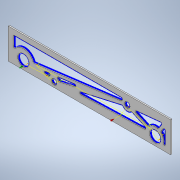
# Autodesk Inventor part: Right right side
Saved by Autodesk Inventor 2021 (Build 250183000, 183)
## iProperties
Created: 2020-09-20
Part Number: Right right side
Material: Generic
Document SubType Name: Modeling
Designer: deli
Density: 1 g/cm^3
Appearance: Default
Author: deli
Autodesk Inventor part; units mm, degrees
ref_plane "YZ Plane" through (0, 0, 0) normal (1, 0, 0) x (0, 1, 0)
ref_plane "XZ Plane" through (0, 0, 0) normal (0, 1, 0) x (-1, 0, 0)
ref_plane "XY Plane" through (0, 0, 0) normal (0, 0, 1) x (1, 0, 0)
sketch "Sketch1" plane through (0, 0, 0) normal (0, 0, 1) x (1, 0, 0)
  line L0 (125.1151, 28.732) -> (166.2826, 33.9736)
  arc A0 (167.3819, 27.7268) -> (166.2826, 33.9736) centre (166.6836, 30.824) ccw
  line L1 (167.3819, 27.7268) -> (129.3518, 19.1523)
  arc A1 (126.0625, 20.4145) -> (129.3518, 19.1523) centre (128.6535, 22.2495) ccw
  arc A2 (126.0625, 20.4145) -> (123.528, 23.1069) centre (115.1699, 12.7) ccw
  arc A3 (125.1151, 28.732) -> (123.528, 23.1069) centre (125.5161, 25.5824) ccw
  line L2 (321.3346, 53.089) -> (381.486, 59.0906)
  arc A4 (384.529, 54.3066) -> (381.486, 59.0906) centre (381.8012, 55.9313) ccw
  line L3 (384.529, 54.3066) -> (377.4306, 42.3884)
  arc A5 (373.8567, 40.9528) -> (377.4306, 42.3884) centre (374.7028, 44.013) ccw
  arc A6 (373.8567, 40.9528) -> (352.4725, 34.4311) centre (368.3, 20.8534) ccw
  arc A7 (348.7058, 33.6279) -> (352.4725, 34.4311) centre (350.0627, 36.4983) ccw
  line L4 (348.7058, 33.6279) -> (320.2929, 47.0593)
  arc A8 (321.3346, 53.089) -> (320.2929, 47.0593) centre (321.6498, 49.9297) ccw
  arc A9 (388.6543, 16.3183) -> (390.525, 12.7) centre (391.7533, 15.6278) ccw
  arc A10 (388.6543, 16.3183) -> (383.3263, 35.3128) centre (368.3, 20.8534) ccw
  arc A11 (382.8862, 39.139) -> (383.3263, 35.3128) centre (385.6141, 37.5143) ccw
  line L5 (382.8862, 39.139) -> (387.7972, 47.3844)
  arc A12 (393.7, 45.7598) -> (387.7972, 47.3844) centre (390.525, 45.7598) ccw
  line L6 (393.7, 45.7598) -> (393.7, 15.875)
  arc A13 (390.525, 12.7) -> (393.7, 15.875) centre (390.525, 15.875) ccw
  line L7 (12.7, 38.8139) -> (12.7, 60.325)
  arc A14 (15.875, 63.5) -> (12.7, 60.325) centre (15.875, 60.325) ccw
  line L8 (15.875, 63.5) -> (282.9805, 63.5)
  arc A15 (285.9117, 59.1048) -> (282.9805, 63.5) centre (282.9805, 60.325) ccw
  arc A16 (285.9117, 59.1048) -> (285.3624, 57.5073) centre (298.2343, 53.975) ccw
  arc A17 (282.7016, 55.1979) -> (285.3624, 57.5073) centre (282.3006, 58.3475) ccw
  line L9 (282.7016, 55.1979) -> (65.3364, 27.5219)
  arc A18 (61.9536, 29.5806) -> (65.3364, 27.5219) centre (64.9353, 30.6715) ccw
  arc A19 (61.9536, 29.5806) -> (18.3444, 36.8183) centre (38.1, 20.8534) ccw
  arc A20 (12.7, 38.8139) -> (18.3444, 36.8183) centre (15.875, 38.8139) ccw
  arc A21 (341.9094, 23.18) -> (343.1641, 29.2238) centre (341.8072, 26.3534) ccw
  line L10 (341.9094, 23.18) -> (181.8296, 18.0238)
  arc A22 (181.0291, 24.2944) -> (181.8296, 18.0238) centre (181.7274, 21.1971) ccw
  line L11 (181.0291, 24.2944) -> (284.0524, 47.5227)
  arc A23 (287.3417, 46.2605) -> (284.0524, 47.5227) centre (284.7507, 44.4255) ccw
  arc A24 (287.3417, 46.2605) -> (307.1824, 44.0709) centre (298.2343, 53.975) ccw
  arc A25 (310.6679, 44.5855) -> (307.1824, 44.0709) centre (309.3109, 41.715) ccw
  line L12 (310.6679, 44.5855) -> (343.1641, 29.2238)
  arc A26 (104.4707, 20.6804) -> (103.4554, 19.0977) centre (115.1699, 12.7) ccw
  arc A27 (100.3348, 17.4622) -> (103.4554, 19.0977) centre (100.6689, 20.6195) ccw
  line L13 (100.3348, 17.4622) -> (92.6169, 18.2787)
  arc A28 (92.5499, 24.5856) -> (92.6169, 18.2787) centre (92.9509, 21.436) ccw
  line L14 (92.5499, 24.5856) -> (101.5246, 25.7283)
  arc A29 (104.4707, 20.6804) -> (101.5246, 25.7283) centre (101.9257, 22.5787) ccw
  circle A30 centre (298.2343, 53.975) radius 6.9977
  circle A31 centre (115.1699, 12.7) radius 6.9977
  circle A32 centre (38.1, 20.8534) radius 14.5034
  circle A33 centre (368.3, 20.8534) radius 14.5034
  line L15 (0, 76.2) -> (0, 0)
  line L16 (0, 0) -> (406.4, 0)
  line L17 (406.4, 76.2) -> (406.4, 0)
  line L18 (0, 76.2) -> (406.4, 76.2)
  point P0 (0, 30.4367)
  constraints: 60 point on circle, 38 end point, 34 centre point
extrude "Extrusion1" add sketch "Sketch1" along normal blind 3.175
body "Solid1"
